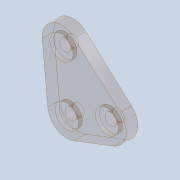
# Autodesk Inventor part: アーム抑え
Saved by Autodesk Inventor 2020.4 (Build 244396000, 396)
## iProperties
Created: 2021-05-06
Part Number: アーム抑え
Material: ポリカーボネート、スモーク
Document SubType Name: Modeling
Designer: happy
Density: 1.2 g/cm^3
Appearance: ポリカーボネート - スモーク
Author: happy
Autodesk Inventor part; units mm, degrees
ref_plane "YZ Plane" through (0, 0, 0) normal (1, 0, 0) x (0, 1, 0)
ref_plane "XZ Plane" through (0, 0, 0) normal (0, 1, 0) x (-1, 0, 0)
ref_plane "XY Plane" through (0, 0, 0) normal (0, 0, 1) x (1, 0, 0)
sketch "スケッチ1" plane through (0, 0, 0) normal (0, 0, 1) x (1, 0, 0)
  circle A0 centre (283.9998, -82.3684) radius 3.025
  circle A1 centre (295.8489, -93.1201) radius 3.025
  circle A2 centre (285.4262, -97.1659) radius 3.025
  circle A3 centre (283.9998, -82.3684) radius 5
  circle A4 centre (295.8489, -93.1201) radius 5
  circle A5 centre (285.4262, -97.1659) radius 5
  line L0 (287.3597, -78.6655) -> (299.2088, -89.4172)
  line L1 (297.6582, -97.7812) -> (287.2355, -101.827)
  line L2 (280.4493, -97.6456) -> (279.0228, -82.8481)
  circle A6 centre (283.9998, -82.3684) radius 1.5
  circle A7 centre (285.4262, -97.1659) radius 1.5
  circle A8 centre (295.8489, -93.1201) radius 1.5
  point P0 (0, 0)
  point P1 (0, 0)
  dimension "d0" = 10
  dimension "d3" = 3
  constraints: 9 centre point, 6 coincident, 6 end point, 6 point on circle, 6 tangent, 4 equal radius, 3 other
  measures "d0" diameter of A3
  measures "d3" diameter of A6
extrude "押し出し1" add sketch "スケッチ1" along normal blind 3 contours A3 | A3 L0 A4 L1 A5 L2 | A4 | A5
extrude "押し出し2" add sketch "スケッチ1" along normal blind 2 contours A0 | A1 | A2
